Autodesk Fusion 360 part; units mm, degrees
(part 6 of 9)
  spline S553 degree 3 poles (-47.1711, -85.1267) (-47.846, -86.0083) (-48.8093, -86.4497) (-50.0598, -86.4497) knots 0 0 0 0 1 1 1 1
  spline S554 degree 3 poles (-50.0598, -86.4497) (-51.2277, -86.4497) (-52.1455, -86.0641) (-52.8142, -85.2921) knots 0 0 0 0 1 1 1 1
  spline S555 degree 3 poles (-52.8142, -85.2921) (-53.4105, -84.548) (-53.7082, -83.6074) (-53.7082, -82.4706) knots 0 0 0 0 1 1 1 1
  spline S556 degree 3 poles (-53.7082, -82.4706) (-53.7082, -81.4443) (-53.4529, -80.5658) (-52.9434, -79.8351) knots 0 0 0 0 1 1 1 1
  spline S557 degree 3 poles (-52.9434, -79.8351) (-52.2892, -78.8977) (-51.3208, -78.4295) (-50.0392, -78.4295) knots 0 0 0 0 1 1 1 1
  spline S558 degree 3 poles (-49.9358, -85.5298) (-49.0294, -85.5298) (-48.3742, -85.2053) (-47.9701, -84.5552) knots 0 0 0 0 1 1 1 1
  spline S559 degree 3 poles (-47.9701, -84.5552) (-47.5649, -83.9061) (-47.3623, -83.1599) (-47.3623, -82.3155) knots 0 0 0 0 1 1 1 1
  spline S560 degree 3 poles (-47.3623, -82.3155) (-47.3623, -81.4236) (-47.5959, -80.7053) (-48.0631, -80.1606) knots 0 0 0 0 1 1 1 1
  spline S561 degree 3 poles (-48.0631, -80.1606) (-48.5292, -79.616) (-49.1679, -79.3441) (-49.9772, -79.3441) knots 0 0 0 0 1 1 1 1
  spline S562 degree 3 poles (-49.9772, -79.3441) (-50.7626, -79.3441) (-51.4034, -79.6139) (-51.8995, -80.1524) knots 0 0 0 0 1 1 1 1
  spline S563 degree 3 poles (-51.8995, -80.1524) (-52.3956, -80.6919) (-52.6437, -81.4866) (-52.6437, -82.5377) knots 0 0 0 0 1 1 1 1
  spline S564 degree 3 poles (-52.6437, -82.5377) (-52.6437, -83.378) (-52.4308, -84.087) (-52.0049, -84.6647) knots 0 0 0 0 1 1 1 1
  spline S565 degree 3 poles (-52.0049, -84.6647) (-51.5802, -85.2415) (-50.8898, -85.5298) (-49.9358, -85.5298) knots 0 0 0 0 1 1 1 1
  line L876 (-49.5224, -76.6311) -> (-48.5561, -76.6311)
  line L877 (-48.5561, -76.6311) -> (-48.5561, -77.706)
  line L878 (-48.5561, -77.706) -> (-49.5224, -77.706)
  line L879 (-49.5224, -77.706) -> (-49.5224, -76.6311)
  line L880 (-51.2277, -76.6311) -> (-50.2614, -76.6311)
  line L881 (-50.2614, -76.6311) -> (-50.2614, -77.706)
  line L882 (-50.2614, -77.706) -> (-51.2277, -77.706)
  line L883 (-51.2277, -77.706) -> (-51.2277, -76.6311)
  line L884 (-35.237, -78.6362) -> (-35.237, -83.3284)
  spline S566 degree 3 poles (-35.237, -83.3284) (-35.237, -83.8793) (-35.1336, -84.3382) (-34.9269, -84.703) knots 0 0 0 0 1 1 1 1
  spline S567 degree 3 poles (-34.9269, -84.703) (-34.62, -85.2539) (-34.1032, -85.5298) (-33.3766, -85.5298) knots 0 0 0 0 1 1 1 1
  spline S568 degree 3 poles (-33.3766, -85.5298) (-32.5054, -85.5298) (-31.9121, -85.2322) (-31.599, -84.6358) knots 0 0 0 0 1 1 1 1
  spline S569 degree 3 poles (-31.599, -84.6358) (-31.4305, -84.3123) (-31.3457, -83.8762) (-31.3457, -83.3284) knots 0 0 0 0 1 1 1 1
  line L885 (-31.3457, -83.3284) -> (-31.3457, -78.6362)
  line L886 (-31.3457, -78.6362) -> (-30.3019, -78.6362)
  line L887 (-30.3019, -78.6362) -> (-30.3019, -82.8995)
  spline S570 degree 3 poles (-30.3019, -82.8995) (-30.3019, -83.8328) (-30.428, -84.5511) (-30.6791, -85.0544) knots 0 0 0 0 1 1 1 1
  spline S571 degree 3 poles (-30.6791, -85.0544) (-31.1411, -85.9711) (-32.0124, -86.429) (-33.2939, -86.429) knots 0 0 0 0 1 1 1 1
  spline S572 degree 3 poles (-33.2939, -86.429) (-34.5755, -86.429) (-35.4458, -85.9711) (-35.9036, -85.0544) knots 0 0 0 0 1 1 1 1
  spline S573 degree 3 poles (-35.9036, -85.0544) (-36.1548, -84.5511) (-36.2808, -83.8328) (-36.2808, -82.8995) knots 0 0 0 0 1 1 1 1
  line L888 (-36.2808, -82.8995) -> (-36.2808, -78.6362)
  line L889 (-36.2808, -78.6362) -> (-35.237, -78.6362)
  line L890 (-18.9971, -78.6362) -> (-13.7313, -78.6362)
  line L891 (-13.7313, -78.6362) -> (-13.7313, -79.5663)
  line L892 (-13.7313, -79.5663) -> (-17.9688, -79.5663)
  line L893 (-17.9688, -79.5663) -> (-17.9688, -81.8711)
  line L894 (-17.9688, -81.8711) -> (-14.2429, -81.8711)
  line L895 (-14.2429, -81.8711) -> (-14.2429, -82.7755)
  line L896 (-14.2429, -82.7755) -> (-17.9688, -82.7755)
  line L897 (-17.9688, -82.7755) -> (-17.9688, -86.2274)
  line L898 (-17.9688, -86.2274) -> (-18.9971, -86.2274)
  line L899 (-18.9971, -86.2274) -> (-18.9971, -78.6362)
  line L900 (-0.4308, -78.6362) -> (0.6079, -78.6362)
  line L901 (0.6079, -78.6362) -> (0.6079, -86.2274)
  line L902 (0.6079, -86.2274) -> (-0.4308, -86.2274)
  line L903 (-0.4308, -86.2274) -> (-0.4308, -78.6362)
  line L904 (14.0437, -78.6362) -> (19.5783, -78.6362)
  line L905 (19.5783, -78.6362) -> (19.5783, -79.5663)
  line L906 (19.5783, -79.5663) -> (15.0463, -79.5663)
  line L907 (15.0463, -79.5663) -> (15.0463, -81.8711)
  line L908 (15.0463, -81.8711) -> (19.2372, -81.8711)
  line L909 (19.2372, -81.8711) -> (19.2372, -82.7496)
  line L910 (19.2372, -82.7496) -> (15.0463, -82.7496)
  line L911 (15.0463, -82.7496) -> (15.0463, -85.3231)
  line L912 (15.0463, -85.3231) -> (19.6558, -85.3231)
  line L913 (19.6558, -85.3231) -> (19.6558, -86.2274)
  line L914 (19.6558, -86.2274) -> (14.0437, -86.2274)
  line L915 (14.0437, -86.2274) -> (14.0437, -78.6362)
  line L916 (30.3218, -78.6362) -> (31.5362, -78.6362)
  line L917 (31.5362, -78.6362) -> (35.3706, -84.7857)
  line L918 (35.3706, -84.7857) -> (35.3706, -78.6362)
  line L919 (35.3706, -78.6362) -> (36.3473, -78.6362)
  line L920 (36.3473, -78.6362) -> (36.3473, -86.2274)
  line L921 (36.3473, -86.2274) -> (35.1949, -86.2274)
  line L922 (35.1949, -86.2274) -> (31.3037, -80.0831)
  line L923 (31.3037, -80.0831) -> (31.3037, -86.2274)
  line L924 (31.3037, -86.2274) -> (30.3218, -86.2274)
  line L925 (30.3218, -86.2274) -> (30.3218, -78.6362)
  line L926 (48.1068, -78.6362) -> (48.1068, -83.3284)
  spline S574 degree 3 poles (48.1068, -83.3284) (48.1068, -83.8793) (48.2101, -84.3382) (48.4168, -84.703) knots 0 0 0 0 1 1 1 1
  spline S575 degree 3 poles (48.4168, -84.703) (48.7238, -85.2539) (49.2406, -85.5298) (49.9671, -85.5298) knots 0 0 0 0 1 1 1 1
  spline S576 degree 3 poles (49.9671, -85.5298) (50.8384, -85.5298) (51.4316, -85.2322) (51.7448, -84.6358) knots 0 0 0 0 1 1 1 1
  spline S577 degree 3 poles (51.7448, -84.6358) (51.9133, -84.3123) (51.998, -83.8762) (51.998, -83.3284) knots 0 0 0 0 1 1 1 1
  line L927 (51.998, -83.3284) -> (51.998, -78.6362)
  line L928 (51.998, -78.6362) -> (53.0419, -78.6362)
  line L929 (53.0419, -78.6362) -> (53.0419, -82.8995)
  spline S578 degree 3 poles (53.0419, -82.8995) (53.0419, -83.8328) (52.9158, -84.5511) (52.6646, -85.0544) knots 0 0 0 0 1 1 1 1
  spline S579 degree 3 poles (52.6646, -85.0544) (52.2026, -85.9711) (51.3314, -86.429) (50.0498, -86.429) knots 0 0 0 0 1 1 1 1
  spline S580 degree 3 poles (50.0498, -86.429) (48.7682, -86.429) (47.898, -85.9711) (47.4401, -85.0544) knots 0 0 0 0 1 1 1 1
  spline S581 degree 3 poles (47.4401, -85.0544) (47.189, -84.5511) (47.0629, -83.8328) (47.0629, -82.8995) knots 0 0 0 0 1 1 1 1
  line L930 (47.0629, -82.8995) -> (47.0629, -78.6362)
  line L931 (47.0629, -78.6362) -> (48.1068, -78.6362)
  line L932 (63.6851, -78.6362) -> (64.7238, -78.6362)
  line L933 (64.7238, -78.6362) -> (64.7238, -81.7729)
  line L934 (64.7238, -81.7729) -> (68.6719, -81.7729)
  line L935 (68.6719, -81.7729) -> (68.6719, -78.6362)
  line L936 (68.6719, -78.6362) -> (69.7106, -78.6362)
  line L937 (69.7106, -78.6362) -> (69.7106, -86.2274)
  line L938 (69.7106, -86.2274) -> (68.6719, -86.2274)
  line L939 (68.6719, -86.2274) -> (68.6719, -82.6773)
  line L940 (68.6719, -82.6773) -> (64.7238, -82.6773)
  line L941 (64.7238, -82.6773) -> (64.7238, -86.2274)
  line L942 (64.7238, -86.2274) -> (63.6851, -86.2274)
  line L943 (63.6851, -86.2274) -> (63.6851, -78.6362)
  spline S582 degree 3 poles (83.8576, -82.114) (84.3402, -82.114) (84.7216, -82.0179) (85.0017, -81.8246) knots 0 0 0 0 1 1 1 1
  spline S583 degree 3 poles (85.0017, -81.8246) (85.2828, -81.6313) (85.4234, -81.2841) (85.4234, -80.7807) knots 0 0 0 0 1 1 1 1
  spline S584 degree 3 poles (85.4234, -80.7807) (85.4234, -80.2402) (85.227, -79.8712) (84.8342, -79.6749) knots 0 0 0 0 1 1 1 1
  spline S585 degree 3 poles (84.8342, -79.6749) (84.6244, -79.5715) (84.3433, -79.5198) (83.9919, -79.5198) knots 0 0 0 0 1 1 1 1
  line L944 (83.9919, -79.5198) -> (81.4804, -79.5198)
  line L945 (81.4804, -79.5198) -> (81.4804, -82.114)
  line L946 (81.4804, -82.114) -> (83.8576, -82.114)
  line L947 (80.4521, -78.6362) -> (83.9661, -78.6362)
  spline S586 degree 3 poles (83.9661, -78.6362) (84.5449, -78.6362) (85.0223, -78.7209) (85.3975, -78.8894) knots 0 0 0 0 1 1 1 1
  spline S587 degree 3 poles (85.3975, -78.8894) (86.1107, -79.2129) (86.4672, -79.8113) (86.4672, -80.6826) knots 0 0 0 0 1 1 1 1
  spline S588 degree 3 poles (86.4672, -80.6826) (86.4672, -81.1373) (86.3732, -81.5094) (86.1861, -81.7988) knots 0 0 0 0 1 1 1 1
  spline S589 degree 3 poles (86.1861, -81.7988) (85.998, -82.0882) (85.7355, -82.3207) (85.3975, -82.4964) knots 0 0 0 0 1 1 1 1
  spline S590 degree 3 poles (85.3975, -82.4964) (85.6941, -82.6173) (85.9174, -82.7755) (86.0662, -82.9718) knots 0 0 0 0 1 1 1 1
  spline S591 degree 3 poles (86.0662, -82.9718) (86.2161, -83.1682) (86.2998, -83.4865) (86.3174, -83.9278) knots 0 0 0 0 1 1 1 1
  line L948 (86.3174, -83.9278) -> (86.3535, -84.9459)
  spline S592 degree 3 poles (86.3535, -84.9459) (86.3639, -85.2353) (86.3876, -85.4502) (86.4259, -85.5918) knots 0 0 0 0 1 1 1 1
  spline S593 degree 3 poles (86.4259, -85.5918) (86.4879, -85.8326) (86.5985, -85.9877) (86.7566, -86.0569) knots 0 0 0 0 1 1 1 1
  line L949 (86.7566, -86.0569) -> (86.7566, -86.2274)
  line L950 (86.7566, -86.2274) -> (85.4957, -86.2274)
  spline S594 degree 3 poles (85.4957, -86.2274) (85.4616, -86.1623) (85.4337, -86.0776) (85.413, -85.9742) knots 0 0 0 0 1 1 1 1
  spline S595 degree 3 poles (85.413, -85.9742) (85.3924, -85.8709) (85.3748, -85.6714) (85.3613, -85.3748) knots 0 0 0 0 1 1 1 1
  line L951 (85.3613, -85.3748) -> (85.2993, -84.1087)
  spline S596 degree 3 poles (85.2993, -84.1087) (85.2756, -83.6126) (85.0906, -83.2798) (84.7464, -83.1114) knots 0 0 0 0 1 1 1 1
  spline S597 degree 3 poles (84.7464, -83.1114) (84.55, -83.0183) (84.242, -82.9718) (83.8214, -82.9718) knots 0 0 0 0 1 1 1 1
  line L952 (83.8214, -82.9718) -> (81.4804, -82.9718)
  line L953 (81.4804, -82.9718) -> (81.4804, -86.2274)
  line L954 (81.4804, -86.2274) -> (80.4521, -86.2274)
  line L955 (80.4521, -86.2274) -> (80.4521, -78.6362)
sketch "Sketch9" plane through (0, 0, 0) normal (0, 0, 1) x (1, 0, 0)
  spline S0 degree 3 poles (105.2213, -98.0075) (105.2213, -99.2498) (104.2146, -100.2575) (102.9713, -100.2575) knots 0 0 0 0 1 1 1 1
  spline S1 degree 3 poles (102.9713, -100.2575) (101.729, -100.2575) (100.7213, -99.2498) (100.7213, -98.0075) knots 0 0 0 0 1 1 1 1
  spline S2 degree 3 poles (100.7213, -98.0075) (100.7213, -96.7652) (101.729, -95.7575) (102.9713, -95.7575) knots 0 0 0 0 1 1 1 1
  spline S3 degree 3 poles (102.9713, -95.7575) (104.2146, -95.7575) (105.2213, -96.7652) (105.2213, -98.0075) knots 0 0 0 0 1 1 1 1
  spline S4 degree 3 poles (105.2213, -98.0075) (105.2213, -99.2498) (104.2136, -100.2575) (102.9713, -100.2575) knots 0 0 0 0 1 1 1 1
  spline S5 degree 3 poles (102.9713, -100.2575) (101.729, -100.2575) (100.7223, -99.2498) (100.7223, -98.0075) knots 0 0 0 0 1 1 1 1
  spline S6 degree 3 poles (100.7223, -98.0075) (100.7223, -96.7652) (101.729, -95.7575) (102.9713, -95.7575) knots 0 0 0 0 1 1 1 1
  spline S7 degree 3 poles (102.9713, -95.7575) (104.2136, -95.7575) (105.2213, -96.7652) (105.2213, -98.0075) knots 0 0 0 0 1 1 1 1
  spline S8 degree 3 poles (-94.7541, -98.0075) (-94.7541, -99.2498) (-95.7618, -100.2575) (-97.0041, -100.2575) knots 0 0 0 0 1 1 1 1
  spline S9 degree 3 poles (-97.0041, -100.2575) (-98.2464, -100.2575) (-99.2541, -99.2498) (-99.2541, -98.0075) knots 0 0 0 0 1 1 1 1
  spline S10 degree 3 poles (-99.2541, -98.0075) (-99.2541, -96.7652) (-98.2464, -95.7575) (-97.0041, -95.7575) knots 0 0 0 0 1 1 1 1
  spline S11 degree 3 poles (-97.0041, -95.7575) (-95.7618, -95.7575) (-94.7541, -96.7652) (-94.7541, -98.0075) knots 0 0 0 0 1 1 1 1
  spline S12 degree 3 poles (-94.7541, -98.0075) (-94.7541, -99.2498) (-95.7618, -100.2575) (-97.0041, -100.2575) knots 0 0 0 0 1 1 1 1
  spline S13 degree 3 poles (-97.0041, -100.2575) (-98.2464, -100.2575) (-99.2541, -99.2498) (-99.2541, -98.0075) knots 0 0 0 0 1 1 1 1
  spline S14 degree 3 poles (-99.2541, -98.0075) (-99.2541, -96.7652) (-98.2464, -95.7575) (-97.0041, -95.7575) knots 0 0 0 0 1 1 1 1
  spline S15 degree 3 poles (-97.0041, -95.7575) (-95.7618, -95.7575) (-94.7541, -96.7652) (-94.7541, -98.0075) knots 0 0 0 0 1 1 1 1
  spline S16 degree 3 poles (-94.7541, 101.9679) (-94.7541, 100.7256) (-95.7618, 99.7179) (-97.0041, 99.7179) knots 0 0 0 0 1 1 1 1
  spline S17 degree 3 poles (-97.0041, 99.7179) (-98.2464, 99.7179) (-99.2541, 100.7256) (-99.2541, 101.9679) knots 0 0 0 0 1 1 1 1
  spline S18 degree 3 poles (-99.2541, 101.9679) (-99.2541, 103.2102) (-98.2464, 104.2179) (-97.0041, 104.2179) knots 0 0 0 0 1 1 1 1
  spline S19 degree 3 poles (-97.0041, 104.2179) (-95.7618, 104.2179) (-94.7541, 103.2102) (-94.7541, 101.9679) knots 0 0 0 0 1 1 1 1
  spline S20 degree 3 poles (-94.7541, 101.9679) (-94.7541, 100.7256) (-95.7618, 99.7179) (-97.0041, 99.7179) knots 0 0 0 0 1 1 1 1
  spline S21 degree 3 poles (-97.0041, 99.7179) (-98.2464, 99.7179) (-99.2541, 100.7256) (-99.2541, 101.9679) knots 0 0 0 0 1 1 1 1
  spline S22 degree 3 poles (-99.2541, 101.9679) (-99.2541, 103.2102) (-98.2464, 104.2179) (-97.0041, 104.2179) knots 0 0 0 0 1 1 1 1
  spline S23 degree 3 poles (-97.0041, 104.2179) (-95.7618, 104.2179) (-94.7541, 103.2102) (-94.7541, 101.9679) knots 0 0 0 0 1 1 1 1
  spline S24 degree 3 poles (105.2213, 101.9679) (105.2213, 100.7256) (104.2146, 99.7179) (102.9713, 99.7179) knots 0 0 0 0 1 1 1 1
  spline S25 degree 3 poles (102.9713, 99.7179) (101.729, 99.7179) (100.7213, 100.7256) (100.7213, 101.9679) knots 0 0 0 0 1 1 1 1
  spline S26 degree 3 poles (100.7213, 101.9679) (100.7213, 103.2102) (101.729, 104.2179) (102.9713, 104.2179) knots 0 0 0 0 1 1 1 1
  spline S27 degree 3 poles (102.9713, 104.2179) (104.2146, 104.2179) (105.2213, 103.2102) (105.2213, 101.9679) knots 0 0 0 0 1 1 1 1
  spline S28 degree 3 poles (105.2213, 101.9679) (105.2213, 100.7256) (104.2136, 99.7179) (102.9713, 99.7179) knots 0 0 0 0 1 1 1 1
  spline S29 degree 3 poles (102.9713, 99.7179) (101.729, 99.7179) (100.7223, 100.7256) (100.7223, 101.9679) knots 0 0 0 0 1 1 1 1
  spline S30 degree 3 poles (100.7223, 101.9679) (100.7223, 103.2102) (101.729, 104.2179) (102.9713, 104.2179) knots 0 0 0 0 1 1 1 1
  spline S31 degree 3 poles (102.9713, 104.2179) (104.2136, 104.2179) (105.2213, 103.2102) (105.2213, 101.9679) knots 0 0 0 0 1 1 1 1
  line L0 (-86.2575, 85.8986) -> (-80.7229, 85.8986)
  line L1 (-80.7229, 85.8986) -> (-80.7229, 84.9684)
  line L2 (-80.7229, 84.9684) -> (-85.2549, 84.9684)
  line L3 (-85.2549, 84.9684) -> (-85.2549, 82.6637)
  line L4 (-85.2549, 82.6637) -> (-81.064, 82.6637)
  line L5 (-81.064, 82.6637) -> (-81.064, 81.7852)
  line L6 (-81.064, 81.7852) -> (-85.2549, 81.7852)
  line L7 (-85.2549, 81.7852) -> (-85.2549, 79.2117)
  line L8 (-85.2549, 79.2117) -> (-80.6454, 79.2117)
  line L9 (-80.6454, 79.2117) -> (-80.6454, 78.3073)
  line L10 (-80.6454, 78.3073) -> (-86.2575, 78.3073)
  line L11 (-86.2575, 78.3073) -> (-86.2575, 85.8986)
  spline S32 degree 3 poles (-69.0151, 80.7568) (-68.9913, 80.3258) (-68.889, 79.9765) (-68.7102, 79.7078) knots 0 0 0 0 1 1 1 1
  spline S33 degree 3 poles (-68.7102, 79.7078) (-68.3691, 79.2044) (-67.7676, 78.9533) (-66.9067, 78.9533) knots 0 0 0 0 1 1 1 1
  spline S34 degree 3 poles (-66.9067, 78.9533) (-66.5212, 78.9533) (-66.1698, 79.0081) (-65.8525, 79.1187) knots 0 0 0 0 1 1 1 1
  spline S35 degree 3 poles (-65.8525, 79.1187) (-65.2396, 79.3326) (-64.9327, 79.715) (-64.9327, 80.2659) knots 0 0 0 0 1 1 1 1
  spline S36 degree 3 poles (-64.9327, 80.2659) (-64.9327, 80.6793) (-65.0618, 80.9738) (-65.3202, 81.1495) knots 0 0 0 0 1 1 1 1
  spline S37 degree 3 poles (-65.3202, 81.1495) (-65.5817, 81.3221) (-65.992, 81.472) (-66.5501, 81.5991) knots 0 0 0 0 1 1 1 1
  line L12 (-66.5501, 81.5991) -> (-67.5785, 81.8317)
  spline S38 degree 3 poles (-67.5785, 81.8317) (-68.2503, 81.9836) (-68.7257, 82.15) (-69.0048, 82.3329) knots 0 0 0 0 1 1 1 1
  spline S39 degree 3 poles (-69.0048, 82.3329) (-69.4874, 82.6502) (-69.7282, 83.1236) (-69.7282, 83.754) knots 0 0 0 0 1 1 1 1
  spline S40 degree 3 poles (-69.7282, 83.754) (-69.7282, 84.4362) (-69.4926, 84.9963) (-69.0203, 85.4335) knots 0 0 0 0 1 1 1 1
  spline S41 degree 3 poles (-69.0203, 85.4335) (-68.5479, 85.8707) (-67.8803, 86.0898) (-67.0152, 86.0898) knots 0 0 0 0 1 1 1 1
  spline S42 degree 3 poles (-67.0152, 86.0898) (-66.2194, 86.0898) (-65.5435, 85.8976) (-64.9864, 85.5131) knots 0 0 0 0 1 1 1 1
  spline S43 degree 3 poles (-64.9864, 85.5131) (-64.4304, 85.1297) (-64.1523, 84.5157) (-64.1523, 83.6714) knots 0 0 0 0 1 1 1 1
  line L13 (-64.1523, 83.6714) -> (-65.1187, 83.6714)
  spline S44 degree 3 poles (-65.1187, 83.6714) (-65.1704, 84.0775) (-65.281, 84.3897) (-65.4494, 84.6067) knots 0 0 0 0 1 1 1 1
  spline S45 degree 3 poles (-65.4494, 84.6067) (-65.7626, 85.0025) (-66.2948, 85.201) (-67.0462, 85.201) knots 0 0 0 0 1 1 1 1
  spline S46 degree 3 poles (-67.0462, 85.201) (-67.6529, 85.201) (-68.088, 85.0739) (-68.3536, 84.8186) knots 0 0 0 0 1 1 1 1
  spline S47 degree 3 poles (-68.3536, 84.8186) (-68.6193, 84.5633) (-68.7515, 84.2677) (-68.7515, 83.9297) knots 0 0 0 0 1 1 1 1
  spline S48 degree 3 poles (-68.7515, 83.9297) (-68.7515, 83.5577) (-68.5965, 83.2858) (-68.2865, 83.1132) knots 0 0 0 0 1 1 1 1
  spline S49 degree 3 poles (-68.2865, 83.1132) (-68.0829, 83.0027) (-67.6229, 82.8652) (-66.9067, 82.6998) knots 0 0 0 0 1 1 1 1
  line L14 (-66.9067, 82.6998) -> (-65.8422, 82.457)
  spline S50 degree 3 poles (-65.8422, 82.457) (-65.3285, 82.3402) (-64.9327, 82.18) (-64.6536, 81.9764) knots 0 0 0 0 1 1 1 1
  spline S51 degree 3 poles (-64.6536, 81.9764) (-64.1709, 81.6219) (-63.9301, 81.1061) (-63.9301, 80.4312) knots 0 0 0 0 1 1 1 1
  spline S52 degree 3 poles (-63.9301, 80.4312) (-63.9301, 79.591) (-64.2361, 78.9895) (-64.8479, 78.6277) knots 0 0 0 0 1 1 1 1
  spline S53 degree 3 poles (-64.8479, 78.6277) (-65.4587, 78.266) (-66.1698, 78.0851) (-66.979, 78.0851) knots 0 0 0 0 1 1 1 1
  spline S54 degree 3 poles (-66.979, 78.0851) (-67.9227, 78.0851) (-68.6616, 78.3259) (-69.196, 78.8086) knots 0 0 0 0 1 1 1 1
  spline S55 degree 3 poles (-69.196, 78.8086) (-69.7303, 79.2871) (-69.9918, 79.9372) (-69.9814, 80.7568) knots 0 0 0 0 1 1 1 1
  line L15 (-69.9814, 80.7568) -> (-69.0151, 80.7568)
  line L16 (-53.0181, 85.8986) -> (-52.0156, 85.8986)
  line L17 (-52.0156, 85.8986) -> (-52.0156, 82.1986)
  line L18 (-52.0156, 82.1986) -> (-48.3156, 85.8986)
  line L19 (-48.3156, 85.8986) -> (-46.8945, 85.8986)
  line L20 (-46.8945, 85.8986) -> (-50.0519, 82.8394)
  line L21 (-50.0519, 82.8394) -> (-46.8066, 78.3073)
  line L22 (-46.8066, 78.3073) -> (-48.1451, 78.3073)
  line L23 (-48.1451, 78.3073) -> (-50.8012, 82.1159)
  line L24 (-50.8012, 82.1159) -> (-52.0156, 80.9532)
  line L25 (-52.0156, 80.9532) -> (-52.0156, 78.3073)
  line L26 (-52.0156, 78.3073) -> (-53.0181, 78.3073)
  line L27 (-53.0181, 78.3073) -> (-53.0181, 85.8986)
  line L28 (-34.057, 85.8986) -> (-33.0183, 85.8986)
  line L29 (-33.0183, 85.8986) -> (-33.0183, 78.3073)
  line L30 (-33.0183, 78.3073) -> (-34.057, 78.3073)
  line L31 (-34.057, 78.3073) -> (-34.057, 85.8986)
  spline S56 degree 3 poles (-19.0088, 80.7568) (-18.9851, 80.3258) (-18.8828, 79.9765) (-18.704, 79.7078) knots 0 0 0 0 1 1 1 1
  spline S57 degree 3 poles (-18.704, 79.7078) (-18.3629, 79.2044) (-17.7614, 78.9533) (-16.9004, 78.9533) knots 0 0 0 0 1 1 1 1
  spline S58 degree 3 poles (-16.9004, 78.9533) (-16.5149, 78.9533) (-16.1635, 79.0081) (-15.8462, 79.1187) knots 0 0 0 0 1 1 1 1
  spline S59 degree 3 poles (-15.8462, 79.1187) (-15.2334, 79.3326) (-14.9264, 79.715) (-14.9264, 80.2659) knots 0 0 0 0 1 1 1 1
  spline S60 degree 3 poles (-14.9264, 80.2659) (-14.9264, 80.6793) (-15.0556, 80.9738) (-15.314, 81.1495) knots 0 0 0 0 1 1 1 1
  spline S61 degree 3 poles (-15.314, 81.1495) (-15.5755, 81.3221) (-15.9858, 81.472) (-16.5439, 81.5991) knots 0 0 0 0 1 1 1 1
  line L32 (-16.5439, 81.5991) -> (-17.5722, 81.8317)
  spline S62 degree 3 poles (-17.5722, 81.8317) (-18.244, 81.9836) (-18.7195, 82.15) (-18.9985, 82.3329) knots 0 0 0 0 1 1 1 1
  spline S63 degree 3 poles (-18.9985, 82.3329) (-19.4812, 82.6502) (-19.722, 83.1236) (-19.722, 83.754) knots 0 0 0 0 1 1 1 1
  spline S64 degree 3 poles (-19.722, 83.754) (-19.722, 84.4362) (-19.4863, 84.9963) (-19.014, 85.4335) knots 0 0 0 0 1 1 1 1
  spline S65 degree 3 poles (-19.014, 85.4335) (-18.5417, 85.8707) (-17.874, 86.0898) (-17.009, 86.0898) knots 0 0 0 0 1 1 1 1
  spline S66 degree 3 poles (-17.009, 86.0898) (-16.2132, 86.0898) (-15.5372, 85.8976) (-14.9802, 85.5131) knots 0 0 0 0 1 1 1 1
  spline S67 degree 3 poles (-14.9802, 85.5131) (-14.4241, 85.1297) (-14.1461, 84.5157) (-14.1461, 83.6714) knots 0 0 0 0 1 1 1 1
  line L33 (-14.1461, 83.6714) -> (-15.1124, 83.6714)
  spline S68 degree 3 poles (-15.1124, 83.6714) (-15.1641, 84.0775) (-15.2747, 84.3897) (-15.4432, 84.6067) knots 0 0 0 0 1 1 1 1
  spline S69 degree 3 poles (-15.4432, 84.6067) (-15.7563, 85.0025) (-16.2886, 85.201) (-17.04, 85.201) knots 0 0 0 0 1 1 1 1
  spline S70 degree 3 poles (-17.04, 85.201) (-17.6467, 85.201) (-18.0818, 85.0739) (-18.3474, 84.8186) knots 0 0 0 0 1 1 1 1
  spline S71 degree 3 poles (-18.3474, 84.8186) (-18.613, 84.5633) (-18.7453, 84.2677) (-18.7453, 83.9297) knots 0 0 0 0 1 1 1 1
  spline S72 degree 3 poles (-18.7453, 83.9297) (-18.7453, 83.5577) (-18.5903, 83.2858) (-18.2802, 83.1132) knots 0 0 0 0 1 1 1 1
  spline S73 degree 3 poles (-18.2802, 83.1132) (-18.0766, 83.0027) (-17.6167, 82.8652) (-16.9004, 82.6998) knots 0 0 0 0 1 1 1 1
  line L34 (-16.9004, 82.6998) -> (-15.8359, 82.457)
  spline S74 degree 3 poles (-15.8359, 82.457) (-15.3222, 82.3402) (-14.9264, 82.18) (-14.6474, 81.9764) knots 0 0 0 0 1 1 1 1
  spline S75 degree 3 poles (-14.6474, 81.9764) (-14.1647, 81.6219) (-13.9239, 81.1061) (-13.9239, 80.4312) knots 0 0 0 0 1 1 1 1
  spline S76 degree 3 poles (-13.9239, 80.4312) (-13.9239, 79.591) (-14.2298, 78.9895) (-14.8417, 78.6277) knots 0 0 0 0 1 1 1 1
  spline S77 degree 3 poles (-14.8417, 78.6277) (-15.4525, 78.266) (-16.1635, 78.0851) (-16.9728, 78.0851) knots 0 0 0 0 1 1 1 1
  spline S78 degree 3 poles (-16.9728, 78.0851) (-17.9164, 78.0851) (-18.6554, 78.3259) (-19.1897, 78.8086) knots 0 0 0 0 1 1 1 1
  spline S79 degree 3 poles (-19.1897, 78.8086) (-19.724, 79.2871) (-19.9855, 79.9372) (-19.9752, 80.7568) knots 0 0 0 0 1 1 1 1
  line L35 (-19.9752, 80.7568) -> (-19.0088, 80.7568)
  line L36 (2.8089, 85.8986) -> (2.8089, 84.9943)
  line L37 (2.8089, 84.9943) -> (0.251, 84.9943)
  line L38 (0.251, 84.9943) -> (0.251, 78.3073)
  line L39 (0.251, 78.3073) -> (-0.7929, 78.3073)
  line L40 (-0.7929, 78.3073) -> (-0.7929, 84.9943)
  line L41 (-0.7929, 84.9943) -> (-3.3509, 84.9943)
  line L42 (-3.3509, 84.9943) -> (-3.3509, 85.8986)
  line L43 (-3.3509, 85.8986) -> (2.8089, 85.8986)
  line L44 (14.2429, 85.8986) -> (15.2712, 85.8986)
  line L45 (15.2712, 85.8986) -> (15.2712, 79.2117)
  line L46 (15.2712, 79.2117) -> (19.116, 79.2117)
  line L47 (19.116, 79.2117) -> (19.116, 78.3073)
  line L48 (19.116, 78.3073) -> (14.2429, 78.3073)
  line L49 (14.2429, 78.3073) -> (14.2429, 85.8986)
  line L50 (30.7204, 85.8986) -> (35.9862, 85.8986)
  line L51 (35.9862, 85.8986) -> (35.9862, 84.9684)
  line L52 (35.9862, 84.9684) -> (31.7488, 84.9684)
  line L53 (31.7488, 84.9684) -> (31.7488, 82.6637)
  line L54 (31.7488, 82.6637) -> (35.4747, 82.6637)
  line L55 (35.4747, 82.6637) -> (35.4747, 81.7593)
  line L56 (35.4747, 81.7593) -> (31.7488, 81.7593)
  line L57 (31.7488, 81.7593) -> (31.7488, 78.3073)
  line L58 (31.7488, 78.3073) -> (30.7204, 78.3073)
  line L59 (30.7204, 78.3073) -> (30.7204, 85.8986)
  line L60 (47.8181, 85.8986) -> (47.8181, 81.2064)
  spline S80 degree 3 poles (47.8181, 81.2064) (47.8181, 80.6555) (47.9214, 80.1966) (48.1281, 79.8318) knots 0 0 0 0 1 1 1 1
  spline S81 degree 3 poles (48.1281, 79.8318) (48.4351, 79.2809) (48.9519, 79.005) (49.6784, 79.005) knots 0 0 0 0 1 1 1 1
  spline S82 degree 3 poles (49.6784, 79.005) (50.5497, 79.005) (51.1429, 79.3026) (51.4561, 79.899) knots 0 0 0 0 1 1 1 1
  spline S83 degree 3 poles (51.4561, 79.899) (51.6246, 80.2225) (51.7093, 80.6586) (51.7093, 81.2064) knots 0 0 0 0 1 1 1 1
  line L61 (51.7093, 81.2064) -> (51.7093, 85.8986)
  line L62 (51.7093, 85.8986) -> (52.7532, 85.8986)
  line L63 (52.7532, 85.8986) -> (52.7532, 81.6353)
  spline S84 degree 3 poles (52.7532, 81.6353) (52.7532, 80.702) (52.6271, 79.9837) (52.3759, 79.4804) knots 0 0 0 0 1 1 1 1
  spline S85 degree 3 poles (52.3759, 79.4804) (51.914, 78.5637) (51.0427, 78.1058) (49.7611, 78.1058) knots 0 0 0 0 1 1 1 1
  spline S86 degree 3 poles (49.7611, 78.1058) (48.4795, 78.1058) (47.6093, 78.5637) (47.1515, 79.4804) knots 0 0 0 0 1 1 1 1
  spline S87 degree 3 poles (47.1515, 79.4804) (46.9003, 79.9837) (46.7742, 80.702) (46.7742, 81.6353) knots 0 0 0 0 1 1 1 1
  line L64 (46.7742, 81.6353) -> (46.7742, 85.8986)
  line L65 (46.7742, 85.8986) -> (47.8181, 85.8986)
  line L66 (50.252, 87.6969) -> (51.2184, 87.6969)
  line L67 (51.2184, 87.6969) -> (51.2184, 86.6221)
  line L68 (51.2184, 86.6221) -> (50.252, 86.6221)
  line L69 (50.252, 86.6221) -> (50.252, 87.6969)
  line L70 (48.5467, 87.6969) -> (49.5131, 87.6969)
  line L71 (49.5131, 87.6969) -> (49.5131, 86.6221)
  line L72 (49.5131, 86.6221) -> (48.5467, 86.6221)
  line L73 (48.5467, 86.6221) -> (48.5467, 87.6969)
  line L74 (63.3706, 85.8986) -> (64.585, 85.8986)
  line L75 (64.585, 85.8986) -> (68.4194, 79.7491)
  line L76 (68.4194, 79.7491) -> (68.4194, 85.8986)
  line L77 (68.4194, 85.8986) -> (69.3961, 85.8986)
  line L78 (69.3961, 85.8986) -> (69.3961, 78.3073)
  line L79 (69.3961, 78.3073) -> (68.2437, 78.3073)
  line L80 (68.2437, 78.3073) -> (64.3525, 84.4517)
  line L81 (64.3525, 84.4517) -> (64.3525, 78.3073)
  line L82 (64.3525, 78.3073) -> (63.3706, 78.3073)
  line L83 (63.3706, 78.3073) -> (63.3706, 85.8986)
  line L84 (80.7267, 85.8986) -> (85.9925, 85.8986)
  line L85 (85.9925, 85.8986) -> (85.9925, 84.9684)
  line L86 (85.9925, 84.9684) -> (81.755, 84.9684)
  line L87 (81.755, 84.9684) -> (81.755, 82.6637)
  line L88 (81.755, 82.6637) -> (85.4809, 82.6637)
  line L89 (85.4809, 82.6637) -> (85.4809, 81.7593)
  line L90 (85.4809, 81.7593) -> (81.755, 81.7593)
  line L91 (81.755, 81.7593) -> (81.755, 78.3073)
  line L92 (81.755, 78.3073) -> (80.7267, 78.3073)
  line L93 (80.7267, 78.3073) -> (80.7267, 85.8986)
  line L94 (-86.6223, 60.6598) -> (-81.9662, 66.4941)
  line L95 (-81.9662, 66.4941) -> (-86.2812, 66.4941)
  line L96 (-86.2812, 66.4941) -> (-86.2812, 67.3984)
  line L97 (-86.2812, 67.3984) -> (-80.6433, 67.3984)
  line L98 (-80.6433, 67.3984) -> (-80.6433, 66.5148)
  line L99 (-80.6433, 66.5148) -> (-85.3252, 60.7115)
  line L100 (-85.3252, 60.7115) -> (-80.6433, 60.7115)
  line L101 (-80.6433, 60.7115) -> (-80.6433, 59.8072)
  line L102 (-80.6433, 59.8072) -> (-86.6223, 59.8072)
  line L103 (-86.6223, 59.8072) -> (-86.6223, 60.6598)
  line L104 (-69.5887, 67.3984) -> (-64.0542, 67.3984)
  line L105 (-64.0542, 67.3984) -> (-64.0542, 66.4683)
  line L106 (-64.0542, 66.4683) -> (-68.5862, 66.4683)
  line L107 (-68.5862, 66.4683) -> (-68.5862, 64.1635)
  line L108 (-68.5862, 64.1635) -> (-64.3952, 64.1635)
  line L109 (-64.3952, 64.1635) -> (-64.3952, 63.285)
  line L110 (-64.3952, 63.285) -> (-68.5862, 63.285)
  line L111 (-68.5862, 63.285) -> (-68.5862, 60.7115)
  line L112 (-68.5862, 60.7115) -> (-63.9766, 60.7115)
  line L113 (-63.9766, 60.7115) -> (-63.9766, 59.8072)
  line L114 (-63.9766, 59.8072) -> (-69.5887, 59.8072)
  line L115 (-69.5887, 59.8072) -> (-69.5887, 67.3984)
  line L116 (-53.2848, 67.3984) -> (-52.2461, 67.3984)
  line L117 (-52.2461, 67.3984) -> (-52.2461, 64.2617)
  line L118 (-52.2461, 64.2617) -> (-48.298, 64.2617)
  line L119 (-48.298, 64.2617) -> (-48.298, 67.3984)
  line L120 (-48.298, 67.3984) -> (-47.2593, 67.3984)
  line L121 (-47.2593, 67.3984) -> (-47.2593, 59.8072)
  line L122 (-47.2593, 59.8072) -> (-48.298, 59.8072)
  line L123 (-48.298, 59.8072) -> (-48.298, 63.3573)
  line L124 (-48.298, 63.3573) -> (-52.2461, 63.3573)
  line L125 (-52.2461, 63.3573) -> (-52.2461, 59.8072)
  line L126 (-52.2461, 59.8072) -> (-53.2848, 59.8072)
  line L127 (-53.2848, 59.8072) -> (-53.2848, 67.3984)
  line L128 (-36.6419, 67.3984) -> (-35.4275, 67.3984)
  line L129 (-35.4275, 67.3984) -> (-31.5931, 61.249)
  line L130 (-31.5931, 61.249) -> (-31.5931, 67.3984)
  line L131 (-31.5931, 67.3984) -> (-30.6164, 67.3984)
  line L132 (-30.6164, 67.3984) -> (-30.6164, 59.8072)
  line L133 (-30.6164, 59.8072) -> (-31.7688, 59.8072)
  line L134 (-31.7688, 59.8072) -> (-35.66, 65.9515)
  line L135 (-35.66, 65.9515) -> (-35.66, 59.8072)
  line L136 (-35.66, 59.8072) -> (-36.6419, 59.8072)
  line L137 (-36.6419, 59.8072) -> (-36.6419, 67.3984)
  line L138 (-19.9473, 60.6598) -> (-15.2912, 66.4941)
  line L139 (-15.2912, 66.4941) -> (-19.6062, 66.4941)
  line L140 (-19.6062, 66.4941) -> (-19.6062, 67.3984)
  line L141 (-19.6062, 67.3984) -> (-13.9683, 67.3984)
  line L142 (-13.9683, 67.3984) -> (-13.9683, 66.5148)
  line L143 (-13.9683, 66.5148) -> (-18.6502, 60.7115)
  line L144 (-18.6502, 60.7115) -> (-13.9683, 60.7115)
  line L145 (-13.9683, 60.7115) -> (-13.9683, 59.8072)
  line L146 (-13.9683, 59.8072) -> (-19.9473, 59.8072)
  line L147 (-19.9473, 59.8072) -> (-19.9473, 60.6598)
  line L148 (-3.9751, 67.3984) -> (-2.5437, 61.2231)
  line L149 (-2.5437, 61.2231) -> (-0.828, 67.3984)
  line L150 (-0.828, 67.3984) -> (0.2882, 67.3984)
  line L151 (0.2882, 67.3984) -> (2.0038, 61.2231)
  line L152 (2.0038, 61.2231) -> (3.4353, 67.3984)
  line L153 (3.4353, 67.3984) -> (4.5618, 67.3984)
  line L154 (4.5618, 67.3984) -> (2.5671, 59.8072)
  line L155 (2.5671, 59.8072) -> (1.4871, 59.8072)
  line L156 (1.4871, 59.8072) -> (-0.2648, 66.1014)
  line L157 (-0.2648, 66.1014) -> (-2.0269, 59.8072)
  line L158 (-2.0269, 59.8072) -> (-3.107, 59.8072)
  line L159 (-3.107, 59.8072) -> (-5.0913, 67.3984)
  line L160 (-5.0913, 67.3984) -> (-3.9751, 67.3984)
  line L161 (17.5533, 62.9181) -> (16.4009, 66.2719)
  line L162 (16.4009, 66.2719) -> (15.1761, 62.9181)
  line L163 (15.1761, 62.9181) -> (17.5533, 62.9181)
  line L164 (15.8634, 67.3984) -> (17.0262, 67.3984)
  line L165 (17.0262, 67.3984) -> (19.7805, 59.8072)
  line L166 (19.7805, 59.8072) -> (18.654, 59.8072)
  line L167 (18.654, 59.8072) -> (17.884, 62.0809)
  line L168 (17.884, 62.0809) -> (14.8816, 62.0809)
  line L169 (14.8816, 62.0809) -> (14.0599, 59.8072)
  line L170 (14.0599, 59.8072) -> (13.0057, 59.8072)
  line L171 (13.0057, 59.8072) -> (15.8634, 67.3984)
  line L172 (30.0331, 67.3984) -> (31.2475, 67.3984)
  line L173 (31.2475, 67.3984) -> (35.0819, 61.249)
  line L174 (35.0819, 61.249) -> (35.0819, 67.3984)
  line L175 (35.0819, 67.3984) -> (36.0586, 67.3984)
  line L176 (36.0586, 67.3984) -> (36.0586, 59.8072)
  line L177 (36.0586, 59.8072) -> (34.9062, 59.8072)
  line L178 (34.9062, 59.8072) -> (31.015, 65.9515)
  line L179 (31.015, 65.9515) -> (31.015, 59.8072)
  line L180 (31.015, 59.8072) -> (30.0331, 59.8072)
  line L181 (30.0331, 59.8072) -> (30.0331, 67.3984)
  line L182 (46.7277, 60.6598) -> (51.3838, 66.4941)
  line L183 (51.3838, 66.4941) -> (47.0688, 66.4941)
  line L184 (47.0688, 66.4941) -> (47.0688, 67.3984)
  line L185 (47.0688, 67.3984) -> (52.7067, 67.3984)
  line L186 (52.7067, 67.3984) -> (52.7067, 66.5148)
  line L187 (52.7067, 66.5148) -> (48.0248, 60.7115)
  line L188 (48.0248, 60.7115) -> (52.7067, 60.7115)
  line L189 (52.7067, 60.7115) -> (52.7067, 59.8072)
  line L190 (52.7067, 59.8072) -> (46.7277, 59.8072)
  line L191 (46.7277, 59.8072) -> (46.7277, 60.6598)
  line L192 (65.9555, 67.3984) -> (66.9942, 67.3984)
  line L193 (66.9942, 67.3984) -> (66.9942, 59.8072)
  line L194 (66.9942, 59.8072) -> (65.9555, 59.8072)
  line L195 (65.9555, 59.8072) -> (65.9555, 67.3984)
  spline S88 degree 3 poles (83.0273, 67.5948) (83.7404, 67.5948) (84.3575, 67.4574) (84.8773, 67.1814) knots 0 0 0 0 1 1 1 1
  spline S89 degree 3 poles (84.8773, 67.1814) (85.6318, 66.7856) (86.0938, 66.091) (86.2622, 65.0988) knots 0 0 0 0 1 1 1 1
  line L196 (86.2622, 65.0988) -> (85.2442, 65.0988)
  spline S90 degree 3 poles (85.2442, 65.0988) (85.1202, 65.6538) (84.8639, 66.058) (84.4742, 66.3101) knots 0 0 0 0 1 1 1 1
  spline S91 degree 3 poles (84.4742, 66.3101) (84.0846, 66.5634) (83.5937, 66.6905) (83.0015, 66.6905) knots 0 0 0 0 1 1 1 1
  spline S92 degree 3 poles (83.0015, 66.6905) (82.2987, 66.6905) (81.7075, 66.4269) (81.2259, 65.8998) knots 0 0 0 0 1 1 1 1
  spline S93 degree 3 poles (81.2259, 65.8998) (80.7453, 65.3727) (80.5055, 64.5872) (80.5055, 63.5434) knots 0 0 0 0 1 1 1 1
  spline S94 degree 3 poles (80.5055, 63.5434) (80.5055, 62.6411) (80.7039, 61.9063) (81.0998, 61.3389) knots 0 0 0 0 1 1 1 1
  spline S95 degree 3 poles (81.0998, 61.3389) (81.4956, 60.7725) (82.1416, 60.4893) (83.0376, 60.4893) knots 0 0 0 0 1 1 1 1
  spline S96 degree 3 poles (83.0376, 60.4893) (83.7229, 60.4893) (84.2913, 60.6877) (84.7399, 61.0867) knots 0 0 0 0 1 1 1 1
  spline S97 degree 3 poles (84.7399, 61.0867) (85.1894, 61.4846) (85.4199, 62.1274) (85.4303, 63.0163) knots 0 0 0 0 1 1 1 1
  line L197 (85.4303, 63.0163) -> (83.0531, 63.0163)
  line L198 (83.0531, 63.0163) -> (83.0531, 63.8689)
  line L199 (83.0531, 63.8689) -> (86.3863, 63.8689)
  line L200 (86.3863, 63.8689) -> (86.3863, 59.8072)
  line L201 (86.3863, 59.8072) -> (85.7248, 59.8072)
  line L202 (85.7248, 59.8072) -> (85.4768, 60.7839)
  spline S98 degree 3 poles (85.4768, 60.7839) (85.1285, 60.4015) (84.8205, 60.1358) (84.5518, 59.988) knots 0 0 0 0 1 1 1 1
  spline S99 degree 3 poles (84.5518, 59.988) (84.1001, 59.7328) (83.5265, 59.6056) (82.8309, 59.6056) knots 0 0 0 0 1 1 1 1
  spline S100 degree 3 poles (82.8309, 59.6056) (81.9318, 59.6056) (81.1587, 59.8971) (80.5107, 60.479) knots 0 0 0 0 1 1 1 1
  spline S101 degree 3 poles (80.5107, 60.479) (79.8048, 61.2097) (79.4513, 62.2122) (79.4513, 63.4865) knots 0 0 0 0 1 1 1 1
  spline S102 degree 3 poles (79.4513, 63.4865) (79.4513, 64.7578) (79.7955, 65.7686) (80.4848, 66.5199) knots 0 0 0 0 1 1 1 1
  spline S103 degree 3 poles (80.4848, 66.5199) (81.139, 67.2362) (81.9865, 67.5948) (83.0273, 67.5948) knots 0 0 0 0 1 1 1 1
  spline S104 degree 3 poles (-83.7336, 42.1865) (-83.3853, 42.1865) (-83.1, 42.2227) (-82.8757, 42.2951) knots 0 0 0 0 1 1 1 1
  spline S105 degree 3 poles (-82.8757, 42.2951) (-82.4758, 42.4294) (-82.1492, 42.6878) (-81.8939, 43.0702) knots 0 0 0 0 1 1 1 1
  spline S106 degree 3 poles (-81.8939, 43.0702) (-81.6903, 43.3772) (-81.5446, 43.7699) (-81.4546, 44.2484) knots 0 0 0 0 1 1 1 1
  spline S107 degree 3 poles (-81.4546, 44.2484) (-81.403, 44.5347) (-81.3771, 44.7993) (-81.3771, 45.0443) knots 0 0 0 0 1 1 1 1
  spline S108 degree 3 poles (-81.3771, 45.0443) (-81.3771, 45.9848) (-81.5642, 46.7155) (-81.9373, 47.2353) knots 0 0 0 0 1 1 1 1
  spline S109 degree 3 poles (-81.9373, 47.2353) (-82.3114, 47.7552) (-82.914, 48.0156) (-83.7439, 48.0156) knots 0 0 0 0 1 1 1 1
  line L203 (-83.7439, 48.0156) -> (-85.5681, 48.0156)
  line L204 (-85.5681, 48.0156) -> (-85.5681, 42.1865)
  line L205 (-85.5681, 42.1865) -> (-83.7336, 42.1865)
  line L206 (-86.6016, 48.8993) -> (-83.5269, 48.8993)
  spline S110 degree 3 poles (-83.5269, 48.8993) (-82.483, 48.8993) (-81.6738, 48.5293) (-81.0981, 47.7883) knots 0 0 0 0 1 1 1 1
  spline S111 degree 3 poles (-81.0981, 47.7883) (-80.5844, 47.1196) (-80.3281, 46.2638) (-80.3281, 45.22) knots 0 0 0 0 1 1 1 1
  spline S112 degree 3 poles (-80.3281, 45.22) (-80.3281, 44.4138) (-80.48, 43.6852) (-80.7829, 43.034) knots 0 0 0 0 1 1 1 1
  spline S113 degree 3 poles (-80.7829, 43.034) (-81.3172, 41.8837) (-82.235, 41.308) (-83.5372, 41.308) knots 0 0 0 0 1 1 1 1
  line L207 (-83.5372, 41.308) -> (-86.6016, 41.308)
  line L208 (-86.6016, 41.308) -> (-86.6016, 48.8993)
  spline S114 degree 3 poles (-66.4499, 45.4215) (-65.9672, 45.4215) (-65.5858, 45.5176) (-65.3058, 45.7109) knots 0 0 0 0 1 1 1 1
  spline S115 degree 3 poles (-65.3058, 45.7109) (-65.0246, 45.9042) (-64.8841, 46.2514) (-64.8841, 46.7547) knots 0 0 0 0 1 1 1 1
  spline S116 degree 3 poles (-64.8841, 46.7547) (-64.8841, 47.2953) (-65.0805, 47.6642) (-65.4732, 47.8606) knots 0 0 0 0 1 1 1 1
  spline S117 degree 3 poles (-65.4732, 47.8606) (-65.683, 47.964) (-65.9641, 48.0156) (-66.3155, 48.0156) knots 0 0 0 0 1 1 1 1
  line L209 (-66.3155, 48.0156) -> (-68.827, 48.0156)
  line L210 (-68.827, 48.0156) -> (-68.827, 45.4215)
  line L211 (-68.827, 45.4215) -> (-66.4499, 45.4215)
  line L212 (-69.8554, 48.8993) -> (-66.3414, 48.8993)
  spline S118 degree 3 poles (-66.3414, 48.8993) (-65.7626, 48.8993) (-65.2851, 48.8146) (-64.9099, 48.6461) knots 0 0 0 0 1 1 1 1
  spline S119 degree 3 poles (-64.9099, 48.6461) (-64.1968, 48.3226) (-63.8402, 47.7242) (-63.8402, 46.8529) knots 0 0 0 0 1 1 1 1
  spline S120 degree 3 poles (-63.8402, 46.8529) (-63.8402, 46.3982) (-63.9343, 46.0261) (-64.1213, 45.7367) knots 0 0 0 0 1 1 1 1
  spline S121 degree 3 poles (-64.1213, 45.7367) (-64.3094, 45.4473) (-64.572, 45.2148) (-64.9099, 45.0391) knots 0 0 0 0 1 1 1 1
  spline S122 degree 3 poles (-64.9099, 45.0391) (-64.6133, 44.9182) (-64.3901, 44.76) (-64.2412, 44.5637) knots 0 0 0 0 1 1 1 1
  spline S123 degree 3 poles (-64.2412, 44.5637) (-64.0914, 44.3673) (-64.0076, 44.049) (-63.9901, 43.6076) knots 0 0 0 0 1 1 1 1
  line L213 (-63.9901, 43.6076) -> (-63.9539, 42.5896)
  spline S124 degree 3 poles (-63.9539, 42.5896) (-63.9436, 42.3002) (-63.9198, 42.0853) (-63.8816, 41.9437) knots 0 0 0 0 1 1 1 1
  spline S125 degree 3 poles (-63.8816, 41.9437) (-63.8195, 41.7029) (-63.709, 41.5478) (-63.5508, 41.4786) knots 0 0 0 0 1 1 1 1
  line L214 (-63.5508, 41.4786) -> (-63.5508, 41.308)
  line L215 (-63.5508, 41.308) -> (-64.8117, 41.308)
  spline S126 degree 3 poles (-64.8117, 41.308) (-64.8458, 41.3732) (-64.8737, 41.4579) (-64.8944, 41.5613) knots 0 0 0 0 1 1 1 1
  spline S127 degree 3 poles (-64.8944, 41.5613) (-64.9151, 41.6646) (-64.9327, 41.8641) (-64.9461, 42.1607) knots 0 0 0 0 1 1 1 1
  line L216 (-64.9461, 42.1607) -> (-65.0081, 43.4268)
  spline S128 degree 3 poles (-65.0081, 43.4268) (-65.0319, 43.9229) (-65.2169, 44.2557) (-65.561, 44.4241) knots 0 0 0 0 1 1 1 1
  spline S129 degree 3 poles (-65.561, 44.4241) (-65.7574, 44.5172) (-66.0654, 44.5637) (-66.4861, 44.5637) knots 0 0 0 0 1 1 1 1
  line L217 (-66.4861, 44.5637) -> (-68.827, 44.5637)
  line L218 (-68.827, 44.5637) -> (-68.827, 41.308)
  line L219 (-68.827, 41.308) -> (-69.8554, 41.308)
  line L220 (-69.8554, 41.308) -> (-69.8554, 48.8993)
  line L221 (-52.92, 48.8993) -> (-47.3854, 48.8993)
  line L222 (-47.3854, 48.8993) -> (-47.3854, 47.9691)
  line L223 (-47.3854, 47.9691) -> (-51.9174, 47.9691)
  line L224 (-51.9174, 47.9691) -> (-51.9174, 45.6644)
  line L225 (-51.9174, 45.6644) -> (-47.7265, 45.6644)
  line L226 (-47.7265, 45.6644) -> (-47.7265, 44.7859)
  line L227 (-47.7265, 44.7859) -> (-51.9174, 44.7859)
  line L228 (-51.9174, 44.7859) -> (-51.9174, 42.2124)
  line L229 (-51.9174, 42.2124) -> (-47.3079, 42.2124)
  line L230 (-47.3079, 42.2124) -> (-47.3079, 41.308)
  line L231 (-47.3079, 41.308) -> (-52.92, 41.308)
  line L232 (-52.92, 41.308) -> (-52.92, 48.8993)
  line L233 (-34.057, 48.8993) -> (-33.0183, 48.8993)
  line L234 (-33.0183, 48.8993) -> (-33.0183, 41.308)
  line L235 (-33.0183, 41.308) -> (-34.057, 41.308)
  line L236 (-34.057, 41.308) -> (-34.057, 48.8993)
  line L237 (-19.0812, 48.8993) -> (-16.9004, 42.4346)
  line L238 (-16.9004, 42.4346) -> (-14.7455, 48.8993)
  line L239 (-14.7455, 48.8993) -> (-13.5932, 48.8993)
  line L240 (-13.5932, 48.8993) -> (-16.363, 41.308)
  line L241 (-16.363, 41.308) -> (-17.4534, 41.308)
  line L242 (-17.4534, 41.308) -> (-20.2181, 48.8993)
  line L243 (-20.2181, 48.8993) -> (-19.0812, 48.8993)
  line L244 (-0.7195, 48.8993) -> (0.3192, 48.8993)
  line L245 (0.3192, 48.8993) -> (0.3192, 41.308)
  line L246 (0.3192, 41.308) -> (-0.7195, 41.308)
  line L247 (-0.7195, 41.308) -> (-0.7195, 48.8993)
  line L248 (13.755, 48.8993) -> (19.2896, 48.8993)
  line L249 (19.2896, 48.8993) -> (19.2896, 47.9691)
  line L250 (19.2896, 47.9691) -> (14.7576, 47.9691)
  line L251 (14.7576, 47.9691) -> (14.7576, 45.6644)
  line L252 (14.7576, 45.6644) -> (18.9485, 45.6644)
  line L253 (18.9485, 45.6644) -> (18.9485, 44.7859)
  line L254 (18.9485, 44.7859) -> (14.7576, 44.7859)
  line L255 (14.7576, 44.7859) -> (14.7576, 42.2124)
  line L256 (14.7576, 42.2124) -> (19.3671, 42.2124)
  line L257 (19.3671, 42.2124) -> (19.3671, 41.308)
  line L258 (19.3671, 41.308) -> (13.755, 41.308)
  line L259 (13.755, 41.308) -> (13.755, 48.8993)
  spline S130 degree 3 poles (33.5626, 45.4215) (34.0453, 45.4215) (34.4267, 45.5176) (34.7067, 45.7109) knots 0 0 0 0 1 1 1 1
  spline S131 degree 3 poles (34.7067, 45.7109) (34.9879, 45.9042) (35.1284, 46.2514) (35.1284, 46.7547) knots 0 0 0 0 1 1 1 1
  spline S132 degree 3 poles (35.1284, 46.7547) (35.1284, 47.2953) (34.932, 47.6642) (34.5393, 47.8606) knots 0 0 0 0 1 1 1 1
  spline S133 degree 3 poles (34.5393, 47.8606) (34.3295, 47.964) (34.0484, 48.0156) (33.697, 48.0156) knots 0 0 0 0 1 1 1 1
  line L260 (33.697, 48.0156) -> (31.1855, 48.0156)
  line L261 (31.1855, 48.0156) -> (31.1855, 45.4215)
  line L262 (31.1855, 45.4215) -> (33.5626, 45.4215)
  line L263 (30.1571, 48.8993) -> (33.6711, 48.8993)
  spline S134 degree 3 poles (33.6711, 48.8993) (34.2499, 48.8993) (34.7274, 48.8146) (35.1026, 48.6461) knots 0 0 0 0 1 1 1 1
  spline S135 degree 3 poles (35.1026, 48.6461) (35.8157, 48.3226) (36.1723, 47.7242) (36.1723, 46.8529) knots 0 0 0 0 1 1 1 1
  spline S136 degree 3 poles (36.1723, 46.8529) (36.1723, 46.3982) (36.0782, 46.0261) (35.8912, 45.7367) knots 0 0 0 0 1 1 1 1
  spline S137 degree 3 poles (35.8912, 45.7367) (35.7031, 45.4473) (35.4405, 45.2148) (35.1026, 45.0391) knots 0 0 0 0 1 1 1 1
  spline S138 degree 3 poles (35.1026, 45.0391) (35.3992, 44.9182) (35.6224, 44.76) (35.7713, 44.5637) knots 0 0 0 0 1 1 1 1
  spline S139 degree 3 poles (35.7713, 44.5637) (35.9211, 44.3673) (36.0049, 44.049) (36.0224, 43.6076) knots 0 0 0 0 1 1 1 1
  line L264 (36.0224, 43.6076) -> (36.0586, 42.5896)
  spline S140 degree 3 poles (36.0586, 42.5896) (36.0689, 42.3002) (36.0927, 42.0853) (36.1309, 41.9437) knots 0 0 0 0 1 1 1 1
  spline S141 degree 3 poles (36.1309, 41.9437) (36.193, 41.7029) (36.3035, 41.5478) (36.4617, 41.4786) knots 0 0 0 0 1 1 1 1
  line L265 (36.4617, 41.4786) -> (36.4617, 41.308)
  line L266 (36.4617, 41.308) -> (35.2008, 41.308)
  spline S142 degree 3 poles (35.2008, 41.308) (35.1667, 41.3732) (35.1388, 41.4579) (35.1181, 41.5613) knots 0 0 0 0 1 1 1 1
  spline S143 degree 3 poles (35.1181, 41.5613) (35.0974, 41.6646) (35.0798, 41.8641) (35.0664, 42.1607) knots 0 0 0 0 1 1 1 1
  line L267 (35.0664, 42.1607) -> (35.0044, 43.4268)
  spline S144 degree 3 poles (35.0044, 43.4268) (34.9806, 43.9229) (34.7956, 44.2557) (34.4515, 44.4241) knots 0 0 0 0 1 1 1 1
  spline S145 degree 3 poles (34.4515, 44.4241) (34.2551, 44.5172) (33.9471, 44.5637) (33.5264, 44.5637) knots 0 0 0 0 1 1 1 1
  line L268 (33.5264, 44.5637) -> (31.1855, 44.5637)
  line L269 (31.1855, 44.5637) -> (31.1855, 41.308)
  line L270 (31.1855, 41.308) -> (30.1571, 41.308)
  line L271 (30.1571, 41.308) -> (30.1571, 48.8993)
  line L272 (52.8152, 48.8993) -> (52.8152, 47.995)
  line L273 (52.8152, 47.995) -> (50.2572, 47.995)
  line L274 (50.2572, 47.995) -> (50.2572, 41.308)
  line L275 (50.2572, 41.308) -> (49.2133, 41.308)
  line L276 (49.2133, 41.308) -> (49.2133, 47.995)
  line L277 (49.2133, 47.995) -> (46.6554, 47.995)
  line L278 (46.6554, 47.995) -> (46.6554, 48.8993)
  line L279 (46.6554, 48.8993) -> (52.8152, 48.8993)
  line L280 (63.7613, 48.8993) -> (69.2958, 48.8993)
  line L281 (69.2958, 48.8993) -> (69.2958, 47.9691)
  line L282 (69.2958, 47.9691) -> (64.7638, 47.9691)
  line L283 (64.7638, 47.9691) -> (64.7638, 45.6644)
  line L284 (64.7638, 45.6644) -> (68.9548, 45.6644)
  line L285 (68.9548, 45.6644) -> (68.9548, 44.7859)
  line L286 (68.9548, 44.7859) -> (64.7638, 44.7859)
  line L287 (64.7638, 44.7859) -> (64.7638, 42.2124)
  line L288 (64.7638, 42.2124) -> (69.3734, 42.2124)
  line L289 (69.3734, 42.2124) -> (69.3734, 41.308)
  line L290 (69.3734, 41.308) -> (63.7613, 41.308)
  line L291 (63.7613, 41.308) -> (63.7613, 48.8993)
  line L292 (80.9179, 48.8993) -> (81.9462, 48.8993)
  line L293 (81.9462, 48.8993) -> (81.9462, 42.2124)
  line L294 (81.9462, 42.2124) -> (85.791, 42.2124)
  line L295 (85.791, 42.2124) -> (85.791, 41.308)
  line L296 (85.791, 41.308) -> (80.9179, 41.308)
  line L297 (80.9179, 41.308) -> (80.9179, 48.8993)
  line L298 (-86.6481, 30.3992) -> (-85.4337, 30.3992)
  line L299 (-85.4337, 30.3992) -> (-81.5993, 24.2497)
  line L300 (-81.5993, 24.2497) -> (-81.5993, 30.3992)
  line L301 (-81.5993, 30.3992) -> (-80.6227, 30.3992)
  line L302 (-80.6227, 30.3992) -> (-80.6227, 22.8079)
  line L303 (-80.6227, 22.8079) -> (-81.775, 22.8079)
  line L304 (-81.775, 22.8079) -> (-85.6663, 28.9522)
  line L305 (-85.6663, 28.9522) -> (-85.6663, 22.8079)
  line L306 (-85.6663, 22.8079) -> (-86.6481, 22.8079)
  line L307 (-86.6481, 22.8079) -> (-86.6481, 30.3992)
  line L308 (-65.7905, 25.9188) -> (-66.9429, 29.2726)
  line L309 (-66.9429, 29.2726) -> (-68.1676, 25.9188)
  line L310 (-68.1676, 25.9188) -> (-65.7905, 25.9188)
  line L311 (-67.4803, 30.3992) -> (-66.3176, 30.3992)
  line L312 (-66.3176, 30.3992) -> (-63.5632, 22.8079)
  line L313 (-63.5632, 22.8079) -> (-64.6898, 22.8079)
  line L314 (-64.6898, 22.8079) -> (-65.4598, 25.0816)
  line L315 (-65.4598, 25.0816) -> (-68.4622, 25.0816)
  line L316 (-68.4622, 25.0816) -> (-69.2838, 22.8079)
  line L317 (-69.2838, 22.8079) -> (-70.338, 22.8079)
  line L318 (-70.338, 22.8079) -> (-67.4803, 30.3992)
  spline S146 degree 3 poles (-50.1119, 30.6059) (-49.1507, 30.6059) (-48.4045, 30.3526) (-47.8743, 29.8462) knots 0 0 0 0 1 1 1 1
  spline S147 degree 3 poles (-47.8743, 29.8462) (-47.3441, 29.3398) (-47.0495, 28.7641) (-46.9906, 28.1202) knots 0 0 0 0 1 1 1 1
  line L319 (-46.9906, 28.1202) -> (-47.9931, 28.1202)
  spline S148 degree 3 poles (-47.9931, 28.1202) (-48.1068, 28.6091) (-48.3332, 28.9967) (-48.6722, 29.2829) knots 0 0 0 0 1 1 1 1
  spline S149 degree 3 poles (-48.6722, 29.2829) (-49.0122, 29.5692) (-49.4886, 29.7119) (-50.1015, 29.7119) knots 0 0 0 0 1 1 1 1
  spline S150 degree 3 poles (-50.1015, 29.7119) (-50.8488, 29.7119) (-51.4523, 29.4493) (-51.9133, 28.9243) knots 0 0 0 0 1 1 1 1
  spline S151 degree 3 poles (-51.9133, 28.9243) (-52.3732, 28.3982) (-52.6027, 27.5931) (-52.6027, 26.5079) knots 0 0 0 0 1 1 1 1
  spline S152 degree 3 poles (-52.6027, 26.5079) (-52.6027, 25.6191) (-52.3949, 24.8977) (-51.9794, 24.3458) knots 0 0 0 0 1 1 1 1
  spline S153 degree 3 poles (-51.9794, 24.3458) (-51.565, 23.7928) (-50.9459, 23.5159) (-50.1222, 23.5159) knots 0 0 0 0 1 1 1 1
  spline S154 degree 3 poles (-50.1222, 23.5159) (-49.3646, 23.5159) (-48.7869, 23.8073) (-48.391, 24.3892) knots 0 0 0 0 1 1 1 1
  spline S155 degree 3 poles (-48.391, 24.3892) (-48.1812, 24.6961) (-48.0241, 25.0992) (-47.9208, 25.5984) knots 0 0 0 0 1 1 1 1
  line L320 (-47.9208, 25.5984) -> (-46.9183, 25.5984)
  spline S156 degree 3 poles (-46.9183, 25.5984) (-47.0082, 24.7995) (-47.3038, 24.1287) (-47.8071, 23.5882) knots 0 0 0 0 1 1 1 1
  spline S157 degree 3 poles (-47.8071, 23.5882) (-48.4096, 22.9371) (-49.223, 22.6115) (-50.2462, 22.6115) knots 0 0 0 0 1 1 1 1
  spline S158 degree 3 poles (-50.2462, 22.6115) (-51.1278, 22.6115) (-51.8689, 22.8782) (-52.4683, 23.4125) knots 0 0 0 0 1 1 1 1
  spline S159 degree 3 poles (-52.4683, 23.4125) (-53.2569, 24.1184) (-53.6517, 25.2088) (-53.6517, 26.6836) knots 0 0 0 0 1 1 1 1
  spline S160 degree 3 poles (-53.6517, 26.6836) (-53.6517, 27.8029) (-53.3551, 28.7217) (-52.7629, 29.438) knots 0 0 0 0 1 1 1 1
  spline S161 degree 3 poles (-52.7629, 29.438) (-52.1221, 30.2162) (-51.2384, 30.6059) (-50.1119, 30.6059) knots 0 0 0 0 1 1 1 1
  line L321 (-36.616, 30.3992) -> (-35.5773, 30.3992)
  line L322 (-35.5773, 30.3992) -> (-35.5773, 27.2624)
  line L323 (-35.5773, 27.2624) -> (-31.6293, 27.2624)
  line L324 (-31.6293, 27.2624) -> (-31.6293, 30.3992)
  line L325 (-31.6293, 30.3992) -> (-30.5906, 30.3992)
  line L326 (-30.5906, 30.3992) -> (-30.5906, 22.8079)
  line L327 (-30.5906, 22.8079) -> (-31.6293, 22.8079)
  line L328 (-31.6293, 22.8079) -> (-31.6293, 26.3581)
  line L329 (-31.6293, 26.3581) -> (-35.5773, 26.3581)
  line L330 (-35.5773, 26.3581) -> (-35.5773, 22.8079)
  line L331 (-35.5773, 22.8079) -> (-36.616, 22.8079)
  line L332 (-36.616, 22.8079) -> (-36.616, 30.3992)
  line L333 (-15.7842, 25.9188) -> (-16.9366, 29.2726)
  line L334 (-16.9366, 29.2726) -> (-18.1614, 25.9188)
  line L335 (-18.1614, 25.9188) -> (-15.7842, 25.9188)
  line L336 (-17.4741, 30.3992) -> (-16.3113, 30.3992)
  line L337 (-16.3113, 30.3992) -> (-13.557, 22.8079)
  line L338 (-13.557, 22.8079) -> (-14.6835, 22.8079)
  line L339 (-14.6835, 22.8079) -> (-15.4535, 25.0816)
  line L340 (-15.4535, 25.0816) -> (-18.4559, 25.0816)
  line L341 (-18.4559, 25.0816) -> (-19.2776, 22.8079)
  line L342 (-19.2776, 22.8079) -> (-20.3318, 22.8079)
  line L343 (-20.3318, 22.8079) -> (-17.4741, 30.3992)
  line L344 (-2.9137, 30.3992) -> (0.5021, 30.3992)
  spline S162 degree 3 poles (0.5021, 30.3992) (1.177, 30.3992) (1.7217, 30.209) (2.1351, 29.8276) knots 0 0 0 0 1 1 1 1